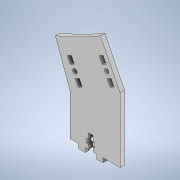
# Autodesk Inventor part: keywell_support-front-r6
Saved by Autodesk Inventor 2020.1 (Build 241239000, 239)
## iProperties
Created: 2019-06-30
Part Number: keywell_support-front-r6
Material: Acier inoxydable
Document SubType Name: Modeling
Designer: Thibault
Density: 8 g/cm^3
Appearance: Semi-poli
Mass: 13.686 g
Surface Area: 39.9351 cm^2
Volume: 1.71076 cm^3
Author: Thibault
Autodesk Inventor part; units mm, degrees
ref_plane "YZ Plane" through (0, 0, 0) normal (1, 0, 0) x (0, 1, 0)
ref_plane "XZ Plane" through (0, 0, 0) normal (0, 1, 0) x (-1, 0, 0)
ref_plane "XY Plane" through (0, 0, 0) normal (0, 0, 1) x (1, 0, 0)
sketch "Anchor (screw side)" plane through (0, 0, 0) normal (0, 0, 1) x (1, 0, 0)
  circle A0 centre (93.7814, 50.2592) radius 1
  line L0 (91.2814, 51.2592) -> (88.2814, 51.2592)
  line L1 (88.2814, 51.2592) -> (88.2814, 49.2592)
  line L2 (88.2814, 49.2592) -> (91.2814, 49.2592)
  line L3 (91.2814, 49.2592) -> (91.2814, 51.2592)
  line L4 (99.2814, 51.2592) -> (96.2814, 51.2592)
  line L5 (96.2814, 51.2592) -> (96.2814, 49.2592)
  line L6 (96.2814, 49.2592) -> (99.2814, 49.2592)
  line L7 (99.2814, 49.2592) -> (99.2814, 51.2592)
  line L8 (91.2814, 51.2592) -> (96.2814, 49.2592) construction
  line L9 (96.2814, 51.2592) -> (91.2814, 49.2592) construction
  line L10 (86.2814, 53.2592) -> (101.2814, 53.2592) construction
  line L11 (101.2814, 53.2592) -> (101.2814, 47.2592) construction
  line L12 (101.2814, 47.2592) -> (86.2814, 47.2592) construction
  line L13 (86.2814, 47.2592) -> (86.2814, 53.2592) construction
  point P0 (103.5798, 50.1132)
  dimension "d27" = 2
  dimension "d28" = 3
  dimension "d29" = 2
  dimension "d30" = 3
  dimension "d32_1" = 5
  dimension "d34" = 2
  dimension "d35" = 2
  dimension "d36" = 2
  dimension "d37" = 2
  measures "d27" diameter of A0
  measures "d28" distance of L2.end L1.end
  measures "d29" distance of L1.end L0.end
  measures "d30" distance of L6.end L5.end
  measures "d32_1" distance between parallel lines of L5 L3
  measures "d34" distance between parallel lines of L0 L10
  measures "d35" distance between parallel lines of L12 L2
  measures "d36" distance between parallel lines of L11 L7
  measures "d37" distance between parallel lines of L13 L1
sketch "Anchor (nut side)" plane through (0, 0, 0) normal (0, 0, 1) x (1, 0, 0)
  line L0 (10, 0) -> (8.5, 0)
  line L1 (8.5, 0) -> (8.5, -2)
  line L2 (8.5, -2) -> (9.3, -2)
  line L3 (9.3, -2) -> (9.3, -4)
  line L4 (5.7, -4) -> (5.7, -2)
  line L5 (5.7, -2) -> (6.5, -2)
  line L6 (6.5, -2) -> (6.5, 0)
  line L7 (6.5, 0) -> (5, 0)
  line L8 (2, 0) -> (2, 2)
  line L9 (2, 0) -> (3, 0) construction
  line L10 (2, 2) -> (5, 2)
  line L11 (5, 2) -> (5, 0)
  line L12 (5, 2) -> (7, 2) construction
  line L13 (10, 0) -> (10, 2)
  line L14 (10, 2) -> (13, 2)
  line L15 (13, 2) -> (13, 0)
  line L16 (0, 0) -> (2, 0)
  line L17 (13, 0) -> (15, 0)
  line L18 (5.7, -4) -> (6.5, -4)
  line L19 (9.3, -4) -> (8.5, -4)
  line L20 (6.5, -4) -> (6.5, -6.25)
  line L21 (8.5, -4) -> (8.5, -6.25)
  line L22 (6.75, -6.5) -> (7.5, -6.5)
  arc A0 (6.5, -6.25) -> (6.75, -6.5) centre (6.75, -6.25) ccw
  arc A1 (8.25, -6.5) -> (8.5, -6.25) centre (8.25, -6.25) ccw
  line L23 (7.5, -7.2938) -> (7.5, -4.9797)
  line L24 (7.5, -6.5) -> (8.25, -6.5)
  point P0 (9.1321, -0.6227)
  point P1 (6.5, -6.5)
  point P2 (8.5, -6.5)
  dimension "d3" = 2
  dimension "d7" = 5
  dimension "d10" = 1.5
  dimension "d11" = 2
  dimension "d12" = 0.8
  dimension "d13" = 2
  dimension "d14" = 0.8
  dimension "d15" = 2
  dimension "d18" = 2
  dimension "d19" = 0.8
  dimension "d20" = 0.8
  dimension "d21" = 2.5
  dimension "d22" = 2.5
  dimension "d23" = 2
  dimension "d38" = 2
  dimension "d39" = 0.25
  dimension "d118" = 2
  dimension "d120" = 3
  measures "d3" distance of point (0, 0) L8.start
  measures "d7" distance of L7.end L0.start
  measures "d10" distance of L0.start L0.end
  measures "d11" distance of L0.end L1.end
  measures "d12" distance of L1.end L2.end
  measures "d13" distance of L2.end L3.end
  measures "d14" distance of L4.end L5.end
  measures "d15" distance of L6.end L0.end
  measures "d18" distance of L15.end point (15, 0)
  measures "d19" distance of L4.start L18.end
  measures "d20" distance of L3.end L19.end
  measures "d21" distance of L18.end point (6.5, -6.5)
  measures "d22" distance of L19.end point (8.5, -6.5)
  measures "d23" distance of L18.end L19.end
  measures "d38" distance of the line from the sketch origin of L10
  measures "d39" radius of A0
  measures "d118" distance between parallel lines of L0 L14
  measures "d120" distance of L8.end L10.end
sketch "Screwless anchor (male)" plane through (0, 0, 0) normal (0, 0, 1) x (1, 0, 0)
  line L0 (1.6, 0) -> (1.6, 2)
  line L1 (1.6, 0) -> (2.6, 0) construction
  line L2 (1.6, 2) -> (4.6, 2)
  line L3 (4.6, 2) -> (4.6, 0)
  line L4 (9.6, 0) -> (9.6, 2)
  line L5 (9.6, 2) -> (12.6, 2)
  line L6 (12.6, 2) -> (12.6, 0)
  line L7 (0, 0) -> (1.6, 0)
  line L8 (12.6, 0) -> (14.2, 0)
  line L9 (4.6, 0) -> (9.6, 0)
  point P0 (9.1321, -0.6227)
  dimension "d81" = 1.6
  dimension "d83" = 5
  dimension "d92" = 1.6
  dimension "d100" = 2
  dimension "d119" = 3
  measures "d81" distance of L7.start L0.start
  measures "d83" distance of L3.end L4.start
  measures "d92" distance of L6.end L8.end
  measures "d100" distance between parallel lines of L7 L2
  measures "d119" distance of L0.end L2.end
sketch "Screwless anchor (female)" plane through (0, 0, 0) normal (0, 0, 1) x (1, 0, 0)
  line L0 (91.2814, 51.2592) -> (88.2814, 51.2592)
  line L1 (88.2814, 51.2592) -> (88.2814, 49.2592)
  line L2 (88.2814, 49.2592) -> (91.2814, 49.2592)
  line L3 (91.2814, 49.2592) -> (91.2814, 51.2592)
  line L4 (99.2814, 51.2592) -> (96.2814, 51.2592)
  line L5 (96.2814, 51.2592) -> (96.2814, 49.2592)
  line L6 (96.2814, 49.2592) -> (99.2814, 49.2592)
  line L7 (99.2814, 49.2592) -> (99.2814, 51.2592)
  line L8 (86.6814, 52.8592) -> (100.8814, 52.8592) construction
  line L9 (100.8814, 52.8592) -> (100.8814, 47.6592) construction
  line L10 (100.8814, 47.6592) -> (86.6814, 47.6592) construction
  line L11 (86.6814, 47.6592) -> (86.6814, 52.8592) construction
  point P0 (103.5798, 50.1132)
  dimension "d106" = 3
  dimension "d107" = 2
  dimension "d108" = 3
  dimension "d109" = 5
  dimension "d110" = 1.6
  dimension "d111" = 1.6
  dimension "d112" = 1.6
  dimension "d113" = 1.6
  measures "d106" distance of L2.end L1.end
  measures "d107" distance of L1.end L0.end
  measures "d108" distance of L6.end L5.end
  measures "d109" distance between parallel lines of L5 L3
  measures "d110" distance between parallel lines of L0 L8
  measures "d111" distance between parallel lines of L10 L2
  measures "d112" distance between parallel lines of L9 L7
  measures "d113" distance between parallel lines of L11 L1
sketch "Anchor" plane through (0, 0, 0) normal (0, 0, 1) x (1, 0, 0)
  line L0 (-55.4359, -124.7421) -> (-44.4359, -138.7421) construction
  line L1 (-44.4359, -124.7421) -> (-55.4359, -138.7421) construction
  line L2 (-49.9359, -129.9428) -> (-49.9359, -133.6158) construction
  circle A0 centre (-49.9359, -123.7421) radius 1
  line L3 (-52.4359, -122.7421) -> (-55.4359, -122.7421)
  line L4 (-55.4359, -122.7421) -> (-55.4359, -124.7421)
  line L5 (-55.4359, -124.7421) -> (-52.4359, -124.7421)
  line L6 (-52.4359, -124.7421) -> (-52.4359, -122.7421)
  line L7 (-44.4359, -122.7421) -> (-47.4359, -122.7421)
  line L8 (-47.4359, -122.7421) -> (-47.4359, -124.7421)
  line L9 (-47.4359, -124.7421) -> (-44.4359, -124.7421)
  line L10 (-44.4359, -124.7421) -> (-44.4359, -122.7421)
  line L11 (-52.4359, -122.7421) -> (-47.4359, -124.7421) construction
  line L12 (-47.4359, -122.7421) -> (-52.4359, -124.7421) construction
  line L13 (-57.4359, -120.7421) -> (-42.4359, -120.7421) construction
  line L14 (-42.4359, -120.7421) -> (-42.4359, -126.7421) construction
  line L15 (-42.4359, -126.7421) -> (-57.4359, -126.7421) construction
  line L16 (-57.4359, -126.7421) -> (-57.4359, -120.7421) construction
  circle A1 centre (-49.9359, -139.7421) radius 1
  line L17 (-52.4359, -138.7421) -> (-55.4359, -138.7421)
  line L18 (-55.4359, -138.7421) -> (-55.4359, -140.7421)
  line L19 (-55.4359, -140.7421) -> (-52.4359, -140.7421)
  line L20 (-52.4359, -140.7421) -> (-52.4359, -138.7421)
  line L21 (-44.4359, -138.7421) -> (-47.4359, -138.7421)
  line L22 (-47.4359, -138.7421) -> (-47.4359, -140.7421)
  line L23 (-47.4359, -140.7421) -> (-44.4359, -140.7421)
  line L24 (-44.4359, -140.7421) -> (-44.4359, -138.7421)
  line L25 (-52.4359, -138.7421) -> (-47.4359, -140.7421) construction
  line L26 (-47.4359, -138.7421) -> (-52.4359, -140.7421) construction
  line L27 (-57.4359, -136.7421) -> (-42.4359, -136.7421) construction
  line L28 (-42.4359, -136.7421) -> (-42.4359, -142.7421) construction
  line L29 (-42.4359, -142.7421) -> (-57.4359, -142.7421) construction
  line L30 (-57.4359, -142.7421) -> (-57.4359, -136.7421) construction
  point P0 (-66.8969, -206.6558)
  point P1 (-49.9359, -123.7421)
  point P2 (-49.9359, -139.7421)
  dimension "d161" = 14
sketch "Esquisse2" plane through (0, 0, 0) normal (0, 0, 1) x (1, 0, 0)
  circle A0 centre (0, 0) radius 190 construction
  arc A1 (-31.3315, -175.2208) -> (89.3705, -153.938) centre (0, 0) ccw
  line L0 (-33.6102, -194.9297) -> (-31.3315, -175.2208)
  line L1 (49.6599, -108.8471) -> (49.6599, -114.6161) construction
  line L2 (98.2525, -171.679) -> (98.2525, -200.8173)
  line L3 (-33.6102, -194.9297) -> (-33.6102, -200.8173)
  line L4 (30.4036, -182.2001) -> (33.7454, -181.6108) construction
  line L5 (89.3705, -153.938) -> (98.2525, -171.679)
  line L6 (-29.3216, -200.8173) -> (-33.6102, -200.8173)
  line L7 (-14.3216, -200.8173) -> (-7.3576, -200.8173)
  line L8 (7.6424, -200.8173) -> (14.6046, -200.8173)
  line L9 (29.6046, -200.8173) -> (37.5335, -200.8173)
  line L10 (52.5335, -200.8173) -> (57.3493, -200.8173)
  line L11 (72.3493, -200.8173) -> (77.5588, -200.8173)
  line L12 (92.5588, -200.8173) -> (98.2525, -200.8173)
  line L13 (28.4172, -182.4328) -> (15.792, -194.9868) construction
  line L14 (29.6969, -193.3581) -> (14.5122, -184.0615) construction
  line L15 (23.8917, -188.5005) -> (20.2437, -188.9278) construction
  circle A2 centre (30.0502, -187.7791) radius 1
  line L16 (30.7526, -185.1797) -> (30.4036, -182.2001)
  line L17 (30.4036, -182.2001) -> (28.4172, -182.4328)
  line L18 (28.4172, -182.4328) -> (28.7662, -185.4124)
  line L19 (28.7662, -185.4124) -> (30.7526, -185.1797)
  line L20 (31.6833, -193.1254) -> (31.3343, -190.1458)
  line L21 (31.3343, -190.1458) -> (29.3479, -190.3784)
  line L22 (29.3479, -190.3784) -> (29.6969, -193.3581)
  line L23 (29.6969, -193.3581) -> (31.6833, -193.1254)
  line L24 (30.7526, -185.1797) -> (29.3479, -190.3784) construction
  line L25 (31.3343, -190.1458) -> (28.7662, -185.4124) construction
  line L26 (32.1573, -179.981) -> (33.9024, -194.8791) construction
  line L27 (33.9024, -194.8791) -> (27.9432, -195.5772) construction
  line L28 (27.9432, -195.5772) -> (26.1981, -180.679) construction
  line L29 (26.1981, -180.679) -> (32.1573, -179.981) construction
  circle A3 centre (14.1589, -189.6405) radius 1
  line L30 (14.8613, -187.0412) -> (14.5122, -184.0615)
  line L31 (14.5122, -184.0615) -> (12.5258, -184.2942)
  line L32 (12.5258, -184.2942) -> (12.8748, -187.2738)
  line L33 (12.8748, -187.2738) -> (14.8613, -187.0412)
  line L34 (15.792, -194.9868) -> (15.443, -192.0072)
  line L35 (15.443, -192.0072) -> (13.4565, -192.2399)
  line L36 (13.4565, -192.2399) -> (13.8056, -195.2195)
  line L37 (13.8056, -195.2195) -> (15.792, -194.9868)
  line L38 (14.8613, -187.0412) -> (13.4565, -192.2399) construction
  line L39 (15.443, -192.0072) -> (12.8748, -187.2738) construction
  line L40 (16.266, -181.8424) -> (18.0111, -196.7406) construction
  line L41 (18.0111, -196.7406) -> (12.0518, -197.4386) construction
  line L42 (12.0518, -197.4386) -> (10.3067, -182.5405) construction
  line L43 (10.3067, -182.5405) -> (16.266, -181.8424) construction
  line L44 (88.8559, -161.8452) -> (81.2616, -177.9489) construction
  line L45 (93.7804, -171.6814) -> (76.3372, -168.1127) construction
  line L46 (86.6678, -169.0915) -> (83.3834, -170.7358) construction
  circle A4 centre (92.2123, -166.3156) radius 1
  line L47 (91.9873, -163.6325) -> (90.6443, -160.9499)
  line L48 (90.6443, -160.9499) -> (88.8559, -161.8452)
  line L49 (88.8559, -161.8452) -> (90.199, -164.5278)
  line L50 (90.199, -164.5278) -> (91.9873, -163.6325)
  line L51 (95.5688, -170.786) -> (94.2257, -168.1034)
  line L52 (94.2257, -168.1034) -> (92.4373, -168.9988)
  line L53 (92.4373, -168.9988) -> (93.7804, -171.6814)
  line L54 (93.7804, -171.6814) -> (95.5688, -170.786)
  line L55 (91.9873, -163.6325) -> (92.4373, -168.9988) construction
  line L56 (94.2257, -168.1034) -> (90.199, -164.5278) construction
  line L57 (91.5373, -158.2661) -> (98.2525, -171.679) construction
  line L58 (98.2525, -171.679) -> (92.8873, -174.3651) construction
  line L59 (92.8873, -174.3651) -> (86.1722, -160.9522) construction
  line L60 (86.1722, -160.9522) -> (91.5373, -158.2661) construction
  circle A5 centre (77.9052, -173.4785) radius 1
  line L61 (77.6802, -170.7953) -> (76.3372, -168.1127)
  line L62 (76.3372, -168.1127) -> (74.5488, -169.0081)
  line L63 (74.5488, -169.0081) -> (75.8918, -171.6906)
  line L64 (75.8918, -171.6906) -> (77.6802, -170.7953)
  line L65 (81.2616, -177.9489) -> (79.9186, -175.2663)
  line L66 (79.9186, -175.2663) -> (78.1302, -176.1616)
  line L67 (78.1302, -176.1616) -> (79.4733, -178.8442)
  line L68 (79.4733, -178.8442) -> (81.2616, -177.9489)
  line L69 (77.6802, -170.7953) -> (78.1302, -176.1616) construction
  line L70 (79.9186, -175.2663) -> (75.8918, -171.6906) construction
  line L71 (77.2302, -165.429) -> (83.9454, -178.8419) construction
  line L72 (83.9454, -178.8419) -> (78.5802, -181.528) construction
  line L73 (78.5802, -181.528) -> (71.8651, -168.115) construction
  line L74 (71.8651, -168.115) -> (77.2302, -165.429) construction
  line L75 (-6.8534, -195.5052) -> (7.1383, -184.4947) construction
  line L76 (-6.8617, -184.5052) -> (7.1466, -195.4947) construction
  line L77 (-1.6569, -190.0013) -> (2.0161, -189.9985) construction
  circle A6 centre (-7.8576, -190.0059) radius 1
  line L78 (-8.8557, -192.5067) -> (-8.8534, -195.5067)
  line L79 (-8.8534, -195.5067) -> (-6.8534, -195.5052)
  line L80 (-6.8534, -195.5052) -> (-6.8557, -192.5052)
  line L81 (-6.8557, -192.5052) -> (-8.8557, -192.5067)
  line L82 (-8.8617, -184.5067) -> (-8.8594, -187.5067)
  line L83 (-8.8594, -187.5067) -> (-6.8594, -187.5052)
  line L84 (-6.8594, -187.5052) -> (-6.8617, -184.5052)
  line L85 (-6.8617, -184.5052) -> (-8.8617, -184.5067)
  line L86 (-8.8557, -192.5067) -> (-6.8594, -187.5052) construction
  line L87 (-8.8594, -187.5067) -> (-6.8557, -192.5052) construction
  line L88 (-10.8519, -197.5082) -> (-10.8632, -182.5082) construction
  line L89 (-10.8632, -182.5082) -> (-4.8632, -182.5037) construction
  line L90 (-4.8632, -182.5037) -> (-4.8519, -197.5037) construction
  line L91 (-4.8519, -197.5037) -> (-10.8519, -197.5082) construction
  circle A7 centre (8.1424, -189.994) radius 1
  line L92 (7.1443, -192.4947) -> (7.1466, -195.4947)
  line L93 (7.1466, -195.4947) -> (9.1466, -195.4932)
  line L94 (9.1466, -195.4932) -> (9.1443, -192.4932)
  line L95 (9.1443, -192.4932) -> (7.1443, -192.4947)
  line L96 (7.1383, -184.4947) -> (7.1406, -187.4947)
  line L97 (7.1406, -187.4947) -> (9.1406, -187.4932)
  line L98 (9.1406, -187.4932) -> (9.1383, -184.4932)
  line L99 (9.1383, -184.4932) -> (7.1383, -184.4947)
  line L100 (7.1443, -192.4947) -> (9.1406, -187.4932) construction
  line L101 (7.1406, -187.4947) -> (9.1443, -192.4932) construction
  line L102 (5.1481, -197.4962) -> (5.1368, -182.4962) construction
  line L103 (5.1368, -182.4962) -> (11.1368, -182.4917) construction
  line L104 (11.1368, -182.4917) -> (11.1481, -197.4917) construction
  line L105 (11.1481, -197.4917) -> (5.1481, -197.4962) construction
  line L106 (-29.407, -193.4024) -> (-14.2363, -184.0831) construction
  line L107 (-28.1436, -182.4752) -> (-15.4996, -195.0103) construction
  line L108 (-23.6091, -188.5361) -> (-19.9604, -188.9579) construction
  circle A8 centre (-29.7687, -187.8239) radius 1
  line L109 (-31.0492, -190.1925) -> (-31.3937, -193.1727)
  line L110 (-31.3937, -193.1727) -> (-29.407, -193.4024)
  line L111 (-29.407, -193.4024) -> (-29.0624, -190.4222)
  line L112 (-29.0624, -190.4222) -> (-31.0492, -190.1925)
  line L113 (-30.1304, -182.2455) -> (-30.4749, -185.2256)
  line L114 (-30.4749, -185.2256) -> (-28.4882, -185.4553)
  line L115 (-28.4882, -185.4553) -> (-28.1436, -182.4752)
  line L116 (-28.1436, -182.4752) -> (-30.1304, -182.2455)
  line L117 (-31.0492, -190.1925) -> (-28.4882, -185.4553) construction
  line L118 (-30.4749, -185.2256) -> (-29.0624, -190.4222) construction
  line L119 (-33.6102, -194.9297) -> (-31.8874, -180.029) construction
  line L120 (-31.8874, -180.029) -> (-25.9271, -180.7181) construction
  line L121 (-25.9271, -180.7181) -> (-27.6499, -195.6188) construction
  line L122 (-27.6499, -195.6188) -> (-33.6102, -194.9297) construction
  circle A9 centre (-13.8746, -189.6615) radius 1
  line L123 (-15.1551, -192.0301) -> (-15.4996, -195.0103)
  line L124 (-15.4996, -195.0103) -> (-13.5128, -195.24)
  line L125 (-13.5128, -195.24) -> (-13.1683, -192.2598)
  line L126 (-13.1683, -192.2598) -> (-15.1551, -192.0301)
  line L127 (-14.2363, -184.0831) -> (-14.5808, -187.0632)
  line L128 (-14.5808, -187.0632) -> (-12.594, -187.2929)
  line L129 (-12.594, -187.2929) -> (-12.2495, -184.3128)
  line L130 (-12.2495, -184.3128) -> (-14.2363, -184.0831)
  line L131 (-15.1551, -192.0301) -> (-12.594, -187.2929) construction
  line L132 (-14.5808, -187.0632) -> (-13.1683, -192.2598) construction
  line L133 (-17.7161, -196.7674) -> (-15.9933, -181.8666) construction
  line L134 (-15.9933, -181.8666) -> (-10.033, -182.5557) construction
  line L135 (-10.033, -182.5557) -> (-11.7558, -197.4565) construction
  line L136 (-11.7558, -197.4565) -> (-17.7161, -196.7674) construction
  line L137 (49.315, -177.9249) -> (38.2257, -191.8542) construction
  line L138 (51.8491, -188.6291) -> (35.6916, -181.1501) construction
  line L139 (45.5213, -184.4751) -> (41.9471, -185.3212) construction
  circle A10 centre (51.5552, -183.0466) radius 1
  line L140 (51.9524, -180.3835) -> (51.2612, -177.4642)
  line L141 (51.2612, -177.4642) -> (49.315, -177.9249)
  line L142 (49.315, -177.9249) -> (50.0061, -180.8442)
  line L143 (50.0061, -180.8442) -> (51.9524, -180.3835)
  line L144 (53.7953, -188.1683) -> (53.1042, -185.249)
  line L145 (53.1042, -185.249) -> (51.158, -185.7097)
  line L146 (51.158, -185.7097) -> (51.8491, -188.6291)
  line L147 (51.8491, -188.6291) -> (53.7953, -188.1683)
  line L148 (51.9524, -180.3835) -> (51.158, -185.7097) construction
  line L149 (53.1042, -185.249) -> (50.0061, -180.8442) construction
  line L150 (52.7467, -175.0572) -> (56.2023, -189.6538) construction
  line L151 (56.2023, -189.6538) -> (50.3636, -191.036) construction
  line L152 (50.3636, -191.036) -> (46.9081, -176.4395) construction
  line L153 (46.9081, -176.4395) -> (52.7467, -175.0572) construction
  circle A11 centre (35.9855, -186.7325) radius 1
  line L154 (36.3827, -184.0694) -> (35.6916, -181.1501)
  line L155 (35.6916, -181.1501) -> (33.7454, -181.6108)
  line L156 (33.7454, -181.6108) -> (34.4365, -184.5302)
  line L157 (34.4365, -184.5302) -> (36.3827, -184.0694)
  line L158 (38.2257, -191.8542) -> (37.5346, -188.9349)
  line L159 (37.5346, -188.9349) -> (35.5883, -189.3957)
  line L160 (35.5883, -189.3957) -> (36.2795, -192.315)
  line L161 (36.2795, -192.315) -> (38.2257, -191.8542)
  line L162 (36.3827, -184.0694) -> (35.5883, -189.3957) construction
  line L163 (37.5346, -188.9349) -> (34.4365, -184.5302) construction
  line L164 (37.1771, -178.7432) -> (40.6326, -193.3397) construction
  line L165 (40.6326, -193.3397) -> (34.794, -194.7219) construction
  line L166 (34.794, -194.7219) -> (31.3384, -180.1254) construction
  line L167 (31.3384, -180.1254) -> (37.1771, -178.7432) construction
  line L168 (69.5517, -171.0316) -> (60.1469, -186.1494) construction
  line L169 (73.3062, -181.371) -> (56.3924, -175.81) construction
  line L170 (66.5406, -177.9764) -> (63.0882, -179.23) construction
  circle A12 centre (72.3689, -175.86) radius 1
  line L171 (72.4556, -173.1688) -> (71.4316, -170.349)
  line L172 (71.4316, -170.349) -> (69.5517, -171.0316)
  line L173 (69.5517, -171.0316) -> (70.5757, -173.8514)
  line L174 (70.5757, -173.8514) -> (72.4556, -173.1688)
  line L175 (75.1861, -180.6884) -> (74.1621, -177.8686)
  line L176 (74.1621, -177.8686) -> (72.2822, -178.5512)
  line L177 (72.2822, -178.5512) -> (73.3062, -181.371)
  line L178 (73.3062, -181.371) -> (75.1861, -180.6884)
  line L179 (72.4556, -173.1688) -> (72.2822, -178.5512) construction
  line L180 (74.1621, -177.8686) -> (70.5757, -173.8514) construction
  line L181 (72.6289, -167.7865) -> (77.7486, -181.8857) construction
  line L182 (77.7486, -181.8857) -> (72.1089, -183.9336) construction
  line L183 (72.1089, -183.9336) -> (66.9892, -169.8343) construction
  line L184 (66.9892, -169.8343) -> (72.6289, -167.7865) construction
  circle A13 centre (57.3297, -181.321) radius 1
  line L185 (57.4164, -178.6298) -> (56.3924, -175.81)
  line L186 (56.3924, -175.81) -> (54.5125, -176.4926)
  line L187 (54.5125, -176.4926) -> (55.5365, -179.3124)
  line L188 (55.5365, -179.3124) -> (57.4164, -178.6298)
  line L189 (60.1469, -186.1494) -> (59.1229, -183.3296)
  line L190 (59.1229, -183.3296) -> (57.243, -184.0122)
  line L191 (57.243, -184.0122) -> (58.267, -186.832)
  line L192 (58.267, -186.832) -> (60.1469, -186.1494)
  line L193 (57.4164, -178.6298) -> (57.243, -184.0122) construction
  line L194 (59.1229, -183.3296) -> (55.5365, -179.3124) construction
  line L195 (57.5897, -173.2474) -> (62.7094, -187.3467) construction
  line L196 (62.7094, -187.3467) -> (57.0697, -189.3946) construction
  line L197 (57.0697, -189.3946) -> (51.95, -175.2953) construction
  line L198 (51.95, -175.2953) -> (57.5897, -173.2474) construction
  line L199 (-24.3216, -200.8173) -> (-22.8216, -200.8173)
  line L200 (-22.8216, -200.8173) -> (-22.8216, -198.8173)
  line L201 (-22.8216, -198.8173) -> (-23.6216, -198.8173)
  line L202 (-23.6216, -198.8173) -> (-23.6216, -196.8173)
  line L203 (-20.0216, -196.8173) -> (-20.0216, -198.8173)
  line L204 (-20.0216, -198.8173) -> (-20.8216, -198.8173)
  line L205 (-20.8216, -198.8173) -> (-20.8216, -200.8173)
  line L206 (-20.8216, -200.8173) -> (-19.3216, -200.8173)
  line L207 (-16.3216, -200.8173) -> (-16.3216, -202.8173)
  line L208 (-16.3216, -200.8173) -> (-17.3216, -200.8173) construction
  line L209 (-16.3216, -202.8173) -> (-19.3216, -202.8173)
  line L210 (-19.3216, -202.8173) -> (-19.3216, -200.8173)
  line L211 (-19.3216, -202.8173) -> (-21.3216, -202.8173) construction
  line L212 (-24.3216, -200.8173) -> (-24.3216, -202.8173)
  line L213 (-24.3216, -202.8173) -> (-27.3216, -202.8173)
  line L214 (-27.3216, -202.8173) -> (-27.3216, -200.8173)
  line L215 (-14.3216, -200.8173) -> (-16.3216, -200.8173)
  line L216 (-27.3216, -200.8173) -> (-29.3216, -200.8173)
  line L217 (-20.0216, -196.8173) -> (-20.8216, -196.8173)
  line L218 (-23.6216, -196.8173) -> (-22.8216, -196.8173)
  line L219 (-20.8216, -196.8173) -> (-20.8216, -194.5673)
  line L220 (-22.8216, -196.8173) -> (-22.8216, -194.5673)
  line L221 (-21.0716, -194.3173) -> (-21.8216, -194.3173)
  arc A14 (-20.8216, -194.5673) -> (-21.0716, -194.3173) centre (-21.0716, -194.5673) ccw
  arc A15 (-22.5716, -194.3173) -> (-22.8216, -194.5673) centre (-22.5716, -194.5673) ccw
  line L222 (-21.8216, -193.5235) -> (-21.8216, -195.8376)
  line L223 (-21.8216, -194.3173) -> (-22.5716, -194.3173)
  line L224 (-2.3576, -200.8173) -> (-0.8576, -200.8173)
  line L225 (-0.8576, -200.8173) -> (-0.8576, -198.8173)
  line L226 (-0.8576, -198.8173) -> (-1.6576, -198.8173)
  line L227 (-1.6576, -198.8173) -> (-1.6576, -196.8173)
  line L228 (1.9424, -196.8173) -> (1.9424, -198.8173)
  line L229 (1.9424, -198.8173) -> (1.1424, -198.8173)
  line L230 (1.1424, -198.8173) -> (1.1424, -200.8173)
  line L231 (1.1424, -200.8173) -> (2.6424, -200.8173)
  line L232 (5.6424, -200.8173) -> (5.6424, -202.8173)
  line L233 (5.6424, -200.8173) -> (4.6424, -200.8173) construction
  line L234 (5.6424, -202.8173) -> (2.6424, -202.8173)
  line L235 (2.6424, -202.8173) -> (2.6424, -200.8173)
  line L236 (2.6424, -202.8173) -> (0.6424, -202.8173) construction
  line L237 (-2.3576, -200.8173) -> (-2.3576, -202.8173)
  line L238 (-2.3576, -202.8173) -> (-5.3576, -202.8173)
  line L239 (-5.3576, -202.8173) -> (-5.3576, -200.8173)
  line L240 (7.6424, -200.8173) -> (5.6424, -200.8173)
  line L241 (-5.3576, -200.8173) -> (-7.3576, -200.8173)
  line L242 (1.9424, -196.8173) -> (1.1424, -196.8173)
  line L243 (-1.6576, -196.8173) -> (-0.8576, -196.8173)
  line L244 (1.1424, -196.8173) -> (1.1424, -194.5673)
  line L245 (-0.8576, -196.8173) -> (-0.8576, -194.5673)
  line L246 (0.8924, -194.3173) -> (0.1424, -194.3173)
  arc A16 (1.1424, -194.5673) -> (0.8924, -194.3173) centre (0.8924, -194.5673) ccw
  arc A17 (-0.6076, -194.3173) -> (-0.8576, -194.5673) centre (-0.6076, -194.5673) ccw
  line L247 (0.1424, -193.5235) -> (0.1424, -195.8376)
  line L248 (0.1424, -194.3173) -> (-0.6076, -194.3173)
  line L249 (19.6046, -200.8173) -> (21.1046, -200.8173)
  line L250 (21.1046, -200.8173) -> (21.1046, -198.8173)
  line L251 (21.1046, -198.8173) -> (20.3046, -198.8173)
  line L252 (20.3046, -198.8173) -> (20.3046, -196.8173)
  line L253 (23.9046, -196.8173) -> (23.9046, -198.8173)
  line L254 (23.9046, -198.8173) -> (23.1046, -198.8173)
  line L255 (23.1046, -198.8173) -> (23.1046, -200.8173)
  line L256 (23.1046, -200.8173) -> (24.6046, -200.8173)
  line L257 (27.6046, -200.8173) -> (27.6046, -202.8173)
  line L258 (27.6046, -200.8173) -> (26.6046, -200.8173) construction
  line L259 (27.6046, -202.8173) -> (24.6046, -202.8173)
  line L260 (24.6046, -202.8173) -> (24.6046, -200.8173)
  line L261 (24.6046, -202.8173) -> (22.6046, -202.8173) construction
  line L262 (19.6046, -200.8173) -> (19.6046, -202.8173)
  line L263 (19.6046, -202.8173) -> (16.6046, -202.8173)
  line L264 (16.6046, -202.8173) -> (16.6046, -200.8173)
  line L265 (29.6046, -200.8173) -> (27.6046, -200.8173)
  line L266 (16.6046, -200.8173) -> (14.6046, -200.8173)
  line L267 (23.9046, -196.8173) -> (23.1046, -196.8173)
  line L268 (20.3046, -196.8173) -> (21.1046, -196.8173)
  line L269 (23.1046, -196.8173) -> (23.1046, -194.5673)
  line L270 (21.1046, -196.8173) -> (21.1046, -194.5673)
  line L271 (22.8546, -194.3173) -> (22.1046, -194.3173)
  arc A18 (23.1046, -194.5673) -> (22.8546, -194.3173) centre (22.8546, -194.5673) ccw
  arc A19 (21.3546, -194.3173) -> (21.1046, -194.5673) centre (21.3546, -194.5673) ccw
  line L272 (22.1046, -193.5235) -> (22.1046, -195.8376)
  line L273 (22.1046, -194.3173) -> (21.3546, -194.3173)
  line L274 (42.5335, -200.8173) -> (44.0335, -200.8173)
  line L275 (44.0335, -200.8173) -> (44.0335, -198.8173)
  line L276 (44.0335, -198.8173) -> (43.2335, -198.8173)
  line L277 (43.2335, -198.8173) -> (43.2335, -196.8173)
  line L278 (46.8335, -196.8173) -> (46.8335, -198.8173)
  line L279 (46.8335, -198.8173) -> (46.0335, -198.8173)
  line L280 (46.0335, -198.8173) -> (46.0335, -200.8173)
  line L281 (46.0335, -200.8173) -> (47.5335, -200.8173)
  line L282 (50.5335, -200.8173) -> (50.5335, -202.8173)
  line L283 (50.5335, -200.8173) -> (49.5335, -200.8173) construction
  line L284 (50.5335, -202.8173) -> (47.5335, -202.8173)
  line L285 (47.5335, -202.8173) -> (47.5335, -200.8173)
  line L286 (47.5335, -202.8173) -> (45.5335, -202.8173) construction
  line L287 (42.5335, -200.8173) -> (42.5335, -202.8173)
  line L288 (42.5335, -202.8173) -> (39.5335, -202.8173)
  line L289 (39.5335, -202.8173) -> (39.5335, -200.8173)
  line L290 (52.5335, -200.8173) -> (50.5335, -200.8173)
  line L291 (39.5335, -200.8173) -> (37.5335, -200.8173)
  line L292 (46.8335, -196.8173) -> (46.0335, -196.8173)
  line L293 (43.2335, -196.8173) -> (44.0335, -196.8173)
  line L294 (46.0335, -196.8173) -> (46.0335, -194.5673)
  line L295 (44.0335, -196.8173) -> (44.0335, -194.5673)
  line L296 (45.7835, -194.3173) -> (45.0335, -194.3173)
  arc A20 (46.0335, -194.5673) -> (45.7835, -194.3173) centre (45.7835, -194.5673) ccw
  arc A21 (44.2835, -194.3173) -> (44.0335, -194.5673) centre (44.2835, -194.5673) ccw
  line L297 (45.0335, -193.5235) -> (45.0335, -195.8376)
  line L298 (45.0335, -194.3173) -> (44.2835, -194.3173)
  line L299 (62.3493, -200.8173) -> (63.8493, -200.8173)
  line L300 (63.8493, -200.8173) -> (63.8493, -198.8173)
  line L301 (63.8493, -198.8173) -> (63.0493, -198.8173)
  line L302 (63.0493, -198.8173) -> (63.0493, -196.8173)
  line L303 (66.6493, -196.8173) -> (66.6493, -198.8173)
  line L304 (66.6493, -198.8173) -> (65.8493, -198.8173)
  line L305 (65.8493, -198.8173) -> (65.8493, -200.8173)
  line L306 (65.8493, -200.8173) -> (67.3493, -200.8173)
  line L307 (70.3493, -200.8173) -> (70.3493, -202.8173)
  line L308 (70.3493, -200.8173) -> (69.3493, -200.8173) construction
  line L309 (70.3493, -202.8173) -> (67.3493, -202.8173)
  line L310 (67.3493, -202.8173) -> (67.3493, -200.8173)
  line L311 (67.3493, -202.8173) -> (65.3493, -202.8173) construction
  line L312 (62.3493, -200.8173) -> (62.3493, -202.8173)
  line L313 (62.3493, -202.8173) -> (59.3493, -202.8173)
  line L314 (59.3493, -202.8173) -> (59.3493, -200.8173)
  line L315 (72.3493, -200.8173) -> (70.3493, -200.8173)
  line L316 (59.3493, -200.8173) -> (57.3493, -200.8173)
  line L317 (66.6493, -196.8173) -> (65.8493, -196.8173)
  line L318 (63.0493, -196.8173) -> (63.8493, -196.8173)
  line L319 (65.8493, -196.8173) -> (65.8493, -194.5673)
  line L320 (63.8493, -196.8173) -> (63.8493, -194.5673)
  line L321 (65.5993, -194.3173) -> (64.8493, -194.3173)
  arc A22 (65.8493, -194.5673) -> (65.5993, -194.3173) centre (65.5993, -194.5673) ccw
  arc A23 (64.0993, -194.3173) -> (63.8493, -194.5673) centre (64.0993, -194.5673) ccw
  line L322 (64.8493, -193.5235) -> (64.8493, -195.8376)
  line L323 (64.8493, -194.3173) -> (64.0993, -194.3173)
  line L324 (82.5588, -200.8173) -> (84.0588, -200.8173)
  line L325 (84.0588, -200.8173) -> (84.0588, -198.8173)
  line L326 (84.0588, -198.8173) -> (83.2588, -198.8173)
  line L327 (83.2588, -198.8173) -> (83.2588, -196.8173)
  line L328 (86.8588, -196.8173) -> (86.8588, -198.8173)
  line L329 (86.8588, -198.8173) -> (86.0588, -198.8173)
  line L330 (86.0588, -198.8173) -> (86.0588, -200.8173)
  line L331 (86.0588, -200.8173) -> (87.5588, -200.8173)
  line L332 (90.5588, -200.8173) -> (90.5588, -202.8173)
  line L333 (90.5588, -200.8173) -> (89.5588, -200.8173) construction
  line L334 (90.5588, -202.8173) -> (87.5588, -202.8173)
  line L335 (87.5588, -202.8173) -> (87.5588, -200.8173)
  line L336 (87.5588, -202.8173) -> (85.5588, -202.8173) construction
  line L337 (82.5588, -200.8173) -> (82.5588, -202.8173)
  line L338 (82.5588, -202.8173) -> (79.5588, -202.8173)
  line L339 (79.5588, -202.8173) -> (79.5588, -200.8173)
  line L340 (92.5588, -200.8173) -> (90.5588, -200.8173)
  line L341 (79.5588, -200.8173) -> (77.5588, -200.8173)
  line L342 (86.8588, -196.8173) -> (86.0588, -196.8173)
  line L343 (83.2588, -196.8173) -> (84.0588, -196.8173)
  line L344 (86.0588, -196.8173) -> (86.0588, -194.5673)
  line L345 (84.0588, -196.8173) -> (84.0588, -194.5673)
  line L346 (85.8088, -194.3173) -> (85.0588, -194.3173)
  arc A24 (86.0588, -194.5673) -> (85.8088, -194.3173) centre (85.8088, -194.5673) ccw
  arc A25 (84.3088, -194.3173) -> (84.0588, -194.5673) centre (84.3088, -194.5673) ccw
  line L347 (85.0588, -193.5235) -> (85.0588, -195.8376)
  line L348 (85.0588, -194.3173) -> (84.3088, -194.3173)
  point P0 (0.1424, -189.9999)
  point P1 (-21.8216, -188.7427)
  point P2 (43.7704, -184.8896)
  point P3 (64.8493, -178.5905)
  point P4 (22.1046, -188.7098)
  point P5 (85.0588, -169.897)
  point P6 (-21.8216, -188.7427)
  point P7 (0.1424, -189.9999)
  point P8 (22.1046, -188.7098)
  point P9 (64.8493, -178.5905)
  point P10 (85.0588, -169.897)
  point P11 (14.6046, -200.8173)
  dimension "radius" = 380
  dimension "d73" = 178
  dimension "d163" = 22
  dimension "d164" = 22
  dimension "d165" = 22
  dimension "d166" = 22
  dimension "d167" = 22
  dimension "d170" = 80
  constraints: 26 end point, 8 point on circle, 7 horizontal, 3 vertical, 2 centre point, 1 coincident, 42 other
  measures "radius" diameter of A0
  measures "d73" radius of A1
  measures "d163" distance of A0.start A0.end
  measures "d164" distance of point (22.105, -188.71) point (43.77, -184.89)
  measures "d165" distance of point (43.77, -184.89) point (64.849, -178.591)
  measures "d166" distance of point (64.849, -178.591) point (85.059, -169.897)
  measures "d167" distance of A0.start point (22.105, -188.71)
  measures "d170" angle of L4 L1
extrude "Base" add sketch "Esquisse2" along normal blind 2
sketch "Esquisse5" plane through (0, 0, 2) normal (0, 0, 1) x (1, 0, 0)
  line L0 (51.0332, -108.3132) -> (187.0726, -108.3132)
  line L1 (187.0726, -108.3132) -> (187.0726, -256.4553)
  line L2 (51.0332, -108.3132) -> (77.7486, -181.8857)
  line L3 (77.7486, -181.8857) -> (77.7486, -256.4553)
  line L4 (77.7486, -256.4553) -> (187.0726, -256.4553)
  line L5 (71.4316, -170.349) -> (72.4556, -173.1688) projected
  line L6 (75.1861, -180.6884) -> (73.3062, -181.371) projected
  point P0 (0, 0)
  dimension "d171" = 2
  dimension "d172" = 2
  constraints: 10 end point, 2 perpendicular, 1 horizontal, 1 parallel, 1 vertical
  measures "d171" distance between parallel lines of L5 L2
  measures "d172" distance from line of L2.end L6
extrude "Front: substract" [suppressed]
sketch "Esquisse7" plane through (0, 0, 2) normal (0, 0, 1) x (1, 0, 0)
  line L0 (75.6984, -182.0982) -> (57.2981, -131.4254)
  line L1 (74.1625, -177.8684) -> (75.1864, -180.6883) projected
  line L2 (-105.9622, -264.9128) -> (-94.3872, -119.3625)
  line L3 (-94.3872, -119.3625) -> (57.2981, -131.4254)
  line L4 (75.6984, -182.0982) -> (75.6984, -264.9128)
  line L5 (75.6984, -264.9128) -> (-105.9622, -264.9128)
  point P0 (0, 0)
  dimension "d156" = 1.5
  constraints: 10 end point, 2 perpendicular, 1 collinear, 1 vertical
  measures "d156" distance of L0.start L1.end
extrude "Front r6: substract" cut sketch "Esquisse7" against normal through all
derived "shared_parameters.ipt"
